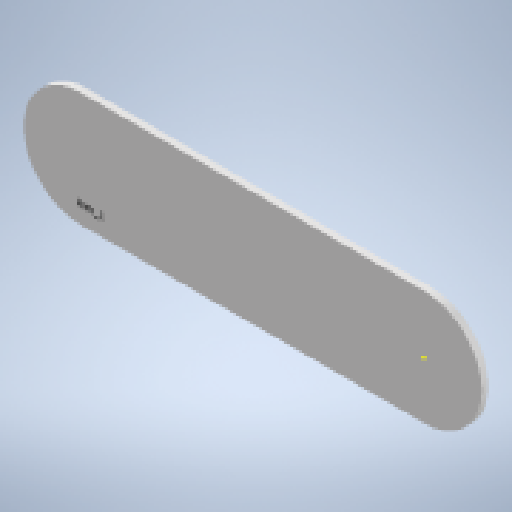
# Autodesk Inventor part: Arm_1
Saved by Autodesk Inventor 2023 (Build 270158000, 158)
## iProperties
Created: 2022-04-08
Part Number: Arm_1
Material: 一般
Document SubType Name: Modeling
Designer: device
Density: 1 g/cm^3
Appearance: 預設
Author: device
Autodesk Inventor part; units mm, degrees
ref_plane "YZ Plane" through (0, 0, 0) normal (1, 0, 0) x (0, 1, 0)
ref_plane "XZ Plane" through (0, 0, 0) normal (0, 1, 0) x (-1, 0, 0)
ref_plane "XY Plane" through (0, 0, 0) normal (0, 0, 1) x (1, 0, 0)
sketch "草圖1" plane through (0, 0, 0) normal (0, 0, 1) x (1, 0, 0)
  line L0 (0, 0) -> (-200, 0) construction
  line L1 (0, 25) -> (-200, 25)
  line L2 (-200, -25) -> (0, -25)
  arc A0 (0, -25) -> (0, 25) centre (0, 0) ccw
  arc A1 (-200, 25) -> (-200, -25) centre (-200, 0) ccw
  point P0 (-100, 0)
  point P1 (25, 0)
  point P2 (-225, 0)
  dimension "d0" = 50
  dimension "d1" = 250
  constraints: 8 end point, 6 point on circle, 4 tangent, 2 centre point, 1 horizontal, 1 midpoint, 1 parallel
  measures "d0" diameter of A1
  measures "d1" distance of point (25, 0) point (-225, 0)
extrude "擠出1" add sketch "草圖1" along normal mid plane 3
sketch "草圖2" plane through (0, 0, 1.5) normal (0, 0, 1) x (1, 0, 0)
  line L0 (-151.7473, -15.3465) -> (-139.1494, -15.3465) construction
  line L1 (-139.1494, -15.3465) -> (-139.1494, -16.9499) construction
  line L2 (-139.1494, -16.9499) -> (-151.7473, -16.9499) construction
  line L3 (-151.7473, -16.9499) -> (-151.7473, -15.3465) construction
  point P0 (0, 0)
  constraints: 2 other
sketch "草圖3" plane through (0, 0, -1.5) normal (0, 0, -1) x (-1, 0, 0)
  circle A0 centre (0, 0) radius 25
  circle A1 centre (0, 0) radius 22
  dimension "d4" = 3
  constraints: 2 centre point, 1 coincident
  measures "d4" radial gap between concentric circles of A0 A1
extrude "擠出2" add sketch "草圖3" along normal blind 44
